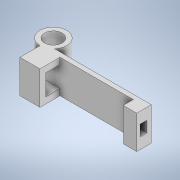
# Autodesk Inventor part: tiny LED's standoff mount
Saved by Autodesk Inventor 2020 (Build 240168000, 168)
## iProperties
Created: 2021-05-09
Part Number: tiny LED's standoff mount
Material: Generic
Document SubType Name: Modeling
Designer: Steven
Density: 1 g/cm^3
Appearance: Default
Author: Steven
Autodesk Inventor part; units mm, degrees
ref_plane "YZ Plane" through (0, 0, 0) normal (1, 0, 0) x (0, 1, 0)
ref_plane "XZ Plane" through (0, 0, 0) normal (0, 1, 0) x (-1, 0, 0)
sketch "Sketch1" plane through (0, 0, 0) normal (0, 1, 0) x (-1, 0, 0)
  circle A0 centre (0, 0) radius 2.625
  circle A1 centre (0, 0) radius 4
  dimension "d0" = 5.25
  dimension "d1" = 8
  constraints: 2 centre point, 2 coincident
  measures "d0" diameter of A0
  measures "d1" diameter of A1
extrude "Extrusion1" add sketch "Sketch1" along normal blind 10
ref_plane "Work Plane1" through (0, 0, 4) normal (0, 0, 1) x (1, 0, 0)
sketch "Sketch2" plane through (0, 0, 4) normal (0, 0, 1) x (1, 0, 0)
  line L0 (4, 10) -> (-4, 10) construction
  line L1 (0, 10) -> (0, 0) construction
  line L2 (0, 10) -> (32, 10)
  line L3 (0, 0) -> (32, 0)
  line L4 (4, 0) -> (-4, 0) projected
  line L5 (0, 10) -> (0, 0)
  line L6 (32, 0) -> (32, 10)
  dimension "d5" = 32
  dimension "d6" = 32
  constraints: 10 end point, 1 collinear, 1 midpoint, 1 perpendicular, 1 point on line, 1 vertical
  measures "d5" distance of L1.start L2.end
  measures "d6" distance of L1.end L3.end
extrude "Extrusion2" add sketch "Sketch2" against normal blind 1.375
sketch "Sketch3" plane through (0, 0, 4) normal (0, 0, 1) x (1, 0, 0)
  line L0 (-2.625, 10) -> (2.625, 10) projected
  line L1 (0, 10) -> (0, 0)
  line L2 (0, 0) -> (6, 0)
  line L3 (32, 0) -> (3.0182, 0) projected
  line L4 (6, 0) -> (6, 10)
  line L5 (6, 10) -> (0, 10)
  dimension "d9" = 6
  constraints: 8 end point, 2 perpendicular, 1 midpoint, 1 point on line, 1 vertical
  measures "d9" distance of L1.end L2.end
extrude "Extrusion3" add sketch "Sketch3" along normal blind 6
sketch "Sketch4" plane through (0, 0, 4) normal (-1, 0, 0) x (0, 0, 1)
  line L0 (6, 0) -> (6, 10) construction
  line L1 (6, 5) -> (0, 5) construction
  line L2 (0, 0) -> (0, 10) construction
  line L3 (0, 5) -> (0, 8.125)
  line L4 (0, 5) -> (0, 1.875)
  line L5 (0, 1.875) -> (4.25, 1.875)
  line L6 (4.25, 1.875) -> (4.25, 8.125)
  line L7 (4.25, 8.125) -> (0, 8.125)
  point P0 (-4, 0)
  dimension "d12" = 3.125
  dimension "d13" = 3.125
  dimension "d14" = 4.25
  constraints: 12 end point, 4 perpendicular, 2 midpoint, 1 point on line
  measures "d12" distance of L1.end L3.end
  measures "d13" distance of L1.end L4.end
  measures "d14" distance of L4.end L5.end
extrude "Extrusion4" cut sketch "Sketch4" against normal up to next
sketch "Sketch5" plane through (0, 0, 4) normal (0, 0, 1) x (1, 0, 0)
  line L0 (32, 10) -> (28, 10)
  line L1 (32, 10) -> (6, 10) projected
  line L2 (28, 10) -> (28, 0)
  line L3 (6, 0) -> (32, 0) projected
  line L4 (32, 0) -> (28, 0)
  line L5 (32, 0) -> (32, 10)
  point P0 (0, 0)
  dimension "d17" = 4
  constraints: 8 end point, 2 point on line, 1 collinear, 1 perpendicular, 1 vertical
  measures "d17" distance of L0.start L0.end
extrude "Extrusion5" add sketch "Sketch5" along normal blind 3
sketch "Sketch6" plane through (28, 0, 4) normal (-1, 0, 0) x (0, 0, 1)
  line L0 (-1.375, 10) -> (3, 10) construction
  line L1 (3, 10) -> (3, 0) construction
  line L2 (0, 0) -> (6, 0) construction
  line L3 (3, 0) -> (3, 10) construction
  line L4 (3, 5) -> (0, 5) construction
  line L5 (0, 1.875) -> (0, 8.125) construction
  line L6 (0, 5) -> (0, 6.625)
  line L7 (0, 5) -> (0, 3.375)
  line L8 (0, 3.375) -> (2, 3.375)
  line L9 (2, 3.375) -> (2, 6.625)
  line L10 (2, 6.625) -> (0, 6.625)
  point P0 (-4, 0)
  dimension "d20" = 1.625
  dimension "d21" = 1.625
  dimension "d22" = 2
  constraints: 14 end point, 3 midpoint, 3 perpendicular, 2 point on line
  measures "d20" distance of L4.end L6.end
  measures "d21" distance of L4.end L7.end
  measures "d22" distance of L7.end L8.end
extrude "Extrusion6" cut sketch "Sketch6" against normal up to next
body "Solid1"
